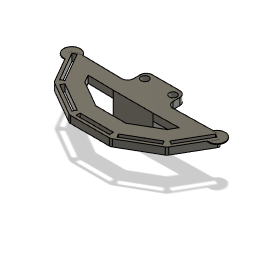
Sensorhållare v11 (Autodesk Fusion 360 design; units mm, degrees)
Autodesk Fusion 360 part; units mm, degrees
note: some values were not read from the file. Set by a fixed rule: which sketch regions a step uses.
sketch "Sketch1" plane through (0, 0, 0) normal (0, 1, 0) x (1, 0, 0)
  line L0 (0, 0) -> (6, 0) construction
  line L1 (0, 0) -> (-6, 0) construction
  circle A0 centre (6, 0) radius 1.6
  circle A1 centre (-6, 0) radius 1.6
  line L2 (0, 0) -> (0, 3) construction
  line L3 (0, 3) -> (-8.4, 3)
  line L4 (-8.4, 3) -> (-8.4, -5)
  line L5 (-8.4, -5) -> (8.4, -5)
  line L6 (8.4, -5) -> (8.4, 3)
  line L7 (8.4, 3) -> (0, 3)
  line L8 (-8, -26.4564) -> (8, -26.4564)
  line L9 (8, -26.4564) -> (21.8564, -18.4564)
  line L10 (-8, -26.4564) -> (-21.8564, -18.4564)
  line L11 (21.8564, -18.4564) -> (8.4, -5) construction
  line L12 (-21.8564, -18.4564) -> (-8.4, -5) construction
  line L13 (21.8564, -18.4564) -> (29.8564, -4.6)
  line L14 (29.8564, -4.6) -> (8.4, -5)
  line L15 (-21.8564, -18.4564) -> (-29.8564, -4.6)
  line L16 (-29.8564, -4.6) -> (-8.4, -5)
  line L17 (-8.4559, -11) -> (8.4559, -11)
  line L18 (19.3504, -10.7969) -> (8.4559, -11)
  line L19 (17.4641, -14.0641) -> (19.3504, -10.7969)
  line L20 (6.3923, -20.4564) -> (17.4641, -14.0641)
  line L21 (-6.3923, -20.4564) -> (6.3923, -20.4564)
  line L22 (-6.3923, -20.4564) -> (-17.4641, -14.0641)
  line L23 (-17.4641, -14.0641) -> (-19.3504, -10.7969)
  line L24 (-19.3504, -10.7969) -> (-8.4559, -11)
  line L25 (-7.1, -28.1064) -> (7.1, -28.1064)
  line L26 (7.1, -26.4564) -> (7.1, -28.1064)
  line L27 (-7.1, -26.4564) -> (-7.1, -28.1064)
  line L28 (-21.077, -18.9064) -> (-21.902, -20.3353)
  line L29 (-21.902, -20.3353) -> (-9.6044, -27.4353)
  line L30 (-9.6044, -27.4353) -> (-8.7794, -26.0064)
  line L31 (-22.3064, -17.677) -> (-23.7353, -18.502)
  line L32 (-23.7353, -18.502) -> (-30.8353, -6.2044)
  line L33 (-30.8353, -6.2044) -> (-29.4064, -5.3794)
  line L34 (29.4064, -5.3794) -> (30.8353, -6.2044)
  line L35 (30.8353, -6.2044) -> (23.7353, -18.502)
  line L36 (23.7353, -18.502) -> (22.3064, -17.677)
  line L37 (8.7794, -26.0064) -> (9.6044, -27.4353)
  line L38 (9.6044, -27.4353) -> (21.902, -20.3353)
  line L39 (21.902, -20.3353) -> (21.077, -18.9064)
  line L40 (0, -28.1064) -> (0, -26.4564) construction
  line L41 (-15.7532, -23.8853) -> (-14.9282, -22.4564) construction
  line L42 (-27.2853, -12.3532) -> (-25.8564, -11.5282) construction
  line L43 (25.8564, -11.5282) -> (27.2853, -12.3532) construction
  line L44 (14.9282, -22.4564) -> (15.7532, -23.8853) construction
  line L45 (23.9794, -20.5794) -> (32.3679, -6.05)
  line L46 (8.7771, -29.3564) -> (23.9794, -20.5794)
  line L47 (-8.7771, -29.3564) -> (8.7771, -29.3564)
  line L48 (-8.7771, -29.3564) -> (-23.9794, -20.5794)
  line L49 (-23.9794, -20.5794) -> (-32.3679, -6.05)
  line L50 (-29.8564, -4.6) -> (-32.3679, -6.05)
  line L51 (32.3679, -6.05) -> (29.8564, -4.6)
  circle A2 centre (6, 0) radius 1.8
  circle A3 centre (-6, 0) radius 1.8
  dimension "d1" = 12
  dimension "d2" = 3.2
  dimension "d4" = 3
  dimension "d5" = 5
  dimension "d7" = 16.8
  dimension "d10" = 135
  dimension "d11" = 135
  dimension "d12" = 30
  dimension "d13" = 16
  dimension "d14" = 26.4564
  dimension "d15" = 60
  dimension "d16" = 6
  dimension "d24" = 14.2
  dimension "d25" = 1.65
  dimension "d26" = -2.9
  dimension "d27" = 3.6
  constraint coincident L0.start L1.start
  constraint horizontal L0
  constraint parallel L0 L1
  constraint equal L0 L1
  constraint coincident L0.end A0.centre
  constraint coincident L1.end A1.centre
  constraint perpendicular L1 L2
  constraint perpendicular L2 L3
  constraint perpendicular L3 L4
  constraint perpendicular L2 L5
  constraint perpendicular L5 L6
  constraint perpendicular L2 L7
  constraint equal L3 L7
  constraint horizontal L8
  constraint equal L11 L12
  constraint equal L9 L10
  constraint equal L8 L9
  constraint equal L14 L16
  constraint equal L13 L15
  constraint equal L10 L15
  constraint horizontal L25
  constraint coincident L8 L26.start
  constraint coincident L8 L27.start
  constraint perpendicular L25 L27
  constraint coincident L10 L28.start
  constraint perpendicular L10 L28
  constraint perpendicular L28 L29
  constraint coincident L10 L30.end
  constraint perpendicular L10 L30
  constraint coincident L15 L31.start
  constraint perpendicular L15 L31
  constraint perpendicular L31 L32
  constraint coincident L15 L33.end
  constraint perpendicular L15 L33
  constraint coincident L13 L34.start
  constraint perpendicular L13 L34
  constraint perpendicular L34 L35
  constraint coincident L13 L36.end
  constraint perpendicular L13 L36
  constraint perpendicular L8 L26
  constraint equal L25 L35
  constraint equal L29 L32
  constraint equal L25 L29
  constraint coincident L9 L37.start
  constraint perpendicular L9 L37
  constraint perpendicular L37 L38
  constraint coincident L9 L39.end
  constraint perpendicular L9 L39
  constraint equal L25 L38
  constraint midpoint L25 L40.start
  constraint midpoint L8 L40.end
  constraint midpoint L29 L41.start
  constraint midpoint L10 L41.end
  constraint midpoint L32 L42.start
  constraint midpoint L15 L42.end
  constraint midpoint L13 L43.start
  constraint midpoint L35 L43.end
  constraint midpoint L9 L44.start
  constraint midpoint L38 L44.end
  constraint perpendicular L13 L43
  constraint perpendicular L9 L44
  constraint perpendicular L8 L40
  constraint perpendicular L10 L41
  constraint perpendicular L15 L42
  constraint equal L27 L33
  constraint equal L27 L28
  constraint equal L27 L37
  constraint equal L27 L36
  constraint perpendicular L13 L51
  constraint concentric A0 A2
  constraint equal A0 A1
  constraint concentric A1 A3
  constraint equal A2 A3
  measures "d1" distance of L0.end L1.end
  measures "d2" diameter of A0
  measures "d4" distance of L0.start L2.end
  measures "d5" distance of L0.start L5
  measures "d7" distance of L4 L6
  measures "d10" angle of L4 L12
  measures "d11" angle of L6 L11
  measures "d12" angle of L5 L9
  measures "d13" distance of L8.start L8.end
  measures "d14" distance of L0.start L8
  measures "d15" angle of L5 L13
  measures "d24" distance of L25.start L25.end
  measures "d25" distance of L25.end L26.start
  measures "d27" diameter of A2
extrude "Extrude1" add sketch "Sketch1" along normal blind 3 contours L3 L4 L5 L6 L7 | L5 L8 L9 L10 L13 L14 L15 L16 | L8 L9 L10 L13 L15 L25 L26 L27 L28 L29 L30 L31 L32 L33 L34 L35 L36 L37 L38 L39 L45 L46 L47 L48 L49 L50 L51 | A2 | A3 makes body 1
sketch "Sketch2" plane through (0, 0, 0) normal (0, -1, 0) x (1, 0, 0)
  line L0 (7.1, 26.4564) -> (-7.1, 26.4564)
  line L1 (-7.1, 26.4564) -> (-7.1, 28.1064)
  line L2 (-7.1, 28.1064) -> (7.1, 28.1064)
  line L3 (7.1, 28.1064) -> (7.1, 26.4564)
  line L4 (8.7794, 26.0064) -> (9.6044, 27.4353)
  line L5 (9.6044, 27.4353) -> (21.902, 20.3353)
  line L6 (21.902, 20.3353) -> (21.077, 18.9064)
  line L7 (21.077, 18.9064) -> (8.7794, 26.0064)
  line L8 (23.7353, 18.502) -> (30.8353, 6.2044)
  line L9 (30.8353, 6.2044) -> (29.4064, 5.3794)
  line L10 (29.4064, 5.3794) -> (22.3064, 17.677)
  line L11 (22.3064, 17.677) -> (23.7353, 18.502)
  line L12 (-22.3064, 17.677) -> (-29.4064, 5.3794)
  line L13 (-29.4064, 5.3794) -> (-30.8353, 6.2044)
  line L14 (-30.8353, 6.2044) -> (-23.7353, 18.502)
  line L15 (-23.7353, 18.502) -> (-22.3064, 17.677)
  circle A0 centre (-6, 0) radius 1.6
  line L16 (-6.3923, 20.4564) -> (6.3923, 20.4564)
  line L17 (6.3923, 20.4564) -> (17.4641, 14.0641)
  line L18 (17.4641, 14.0641) -> (19.3504, 10.7969)
  line L19 (19.3504, 10.7969) -> (8.4559, 11)
  line L20 (8.4559, 11) -> (-8.4559, 11)
  line L21 (-8.4559, 11) -> (-19.3504, 10.7969)
  line L22 (-19.3504, 10.7969) -> (-17.4641, 14.0641)
  line L23 (-17.4641, 14.0641) -> (-6.3923, 20.4564)
  circle A1 centre (6, 0) radius 1.6
  line L24 (-9.6044, 27.4353) -> (-8.7794, 26.0064)
  line L25 (-8.7794, 26.0064) -> (-21.077, 18.9064)
  line L26 (-21.077, 18.9064) -> (-21.902, 20.3353)
  line L27 (-21.902, 20.3353) -> (-9.6044, 27.4353)
  line L28 (8.7771, 29.3564) -> (-8.7771, 29.3564)
  line L29 (-8.7771, 29.3564) -> (-23.9794, 20.5794)
  line L30 (-23.9794, 20.5794) -> (-32.3679, 6.05)
  line L31 (-32.3679, 6.05) -> (-29.8564, 4.6)
  line L32 (-29.8564, 4.6) -> (-8.4, 5)
  line L33 (-8.4, 5) -> (-8.4, -3)
  line L34 (-8.4, -3) -> (8.4, -3)
  line L35 (8.4, -3) -> (8.4, 5)
  line L36 (8.4, 5) -> (29.8564, 4.6)
  line L37 (29.8564, 4.6) -> (32.3679, 6.05)
  line L38 (32.3679, 6.05) -> (23.9794, 20.5794)
  line L39 (23.9794, 20.5794) -> (8.7771, 29.3564)
  line L40 (8.4, 5) -> (8.4559, 11)
  line L41 (-8.4, 5) -> (-8.4559, 11)
  line L42 (-8.4, -1.8) -> (8.4, -1.8)
  circle A2 centre (6, 0) radius 1.8
  circle A3 centre (-6, 0) radius 1.8
  line L43 (8.4, -0.4) -> (-8.4, -0.4)
  line L44 (3.4, -1.8) -> (3.4, -0.4)
  line L45 (-3.4, -1.8) -> (-3.4, -0.4)
  line L46 (8.4, 5) -> (8.4, -3)
  line L47 (-8.4, -3) -> (-8.4, 5)
  line L48 (-8.4, 5) -> (8.4, 5)
  dimension "d28" = 0.4
  dimension "d29" = 5
  dimension "d30" = 5
  constraint coincident L35.end L36.start
  constraint coincident L19.end L20.start
  constraint coincident L32.end L33.start
  constraint coincident L20.end L21.start
  constraint coincident L33 L42.start
  constraint coincident L35 L42.end
  constraint perpendicular L35 L42
  constraint tangent L42 A2
  constraint coincident L35 L43.start
  constraint coincident L33 L43.end
  constraint perpendicular L33 L43
  constraint coincident L42 L44.start
  constraint coincident L43 L44.end
  constraint perpendicular L43 L44
  constraint coincident L42 L45.start
  constraint coincident L43 L45.end
  constraint perpendicular L43 L45
  measures "d28" distance of L43 origin
  measures "d29" distance of L44 L46
  measures "d30" distance of L45 L47
extrude "Extrude4" add sketch "Sketch2" along normal blind 6.2 and the other way blind -4.2 separate body contours A0 A3 L43 | L33 L35 A2 A3 L43 L46 L47 L48 | A1 A2 L43 picked at (-7.7136, -0.2359) picked at (4.2864, -0.2359) makes body 2
extrude "Extrude5" add sketch "Sketch2" along normal blind 11.2 and the other way blind -6.2 separate body contours A0 A3 L43 | L33 L35 A2 A3 L43 L46 L47 L48 | A1 A2 L43 picked at (-7.7136, -0.2359) picked at (4.2864, -0.2359) makes body 3
extrude "Extrude6" add sketch "Sketch2" along normal blind 14.2 and the other way blind -11.2 contours A0 A3 L43 | A0 A3 L43 | L33 L35 A2 A3 L43 L46 L47 L48 | L33 L42 A3 L43 L47 | L42 A3 L43 L45 | L33 L34 L35 L42 L46 L47 | L42 L43 L44 L45 | L42 A2 L43 L44 | A1 A2 L43 | A1 A2 L43 | L35 L42 A2 L43 L46 bodies 3
extrude "Extrude7" add sketch "Sketch2" along normal blind 14.2 contours L20 L40 L41 L48 bodies 1 2 3
sketch "Sketch3" plane through (0, -14.2, 0) normal (0, -1, 0) x (1, 0, 0)
  circle A0 centre (-6, 0) radius 1.6
  circle A1 centre (6, 0) radius 1.6
  line L0 (8.4, 5) -> (8.4559, 11)
  line L1 (8.4559, 11) -> (-8.4559, 11)
  line L2 (-8.4559, 11) -> (-8.4, 5)
  line L3 (-8.4, 5) -> (-8.4, -3)
  line L4 (-8.4, -3) -> (8.4, -3)
  line L5 (8.4, -3) -> (8.4, 5)
  line L6 (-7.6166, 2.8) -> (-9.2332, 0)
  line L7 (-9.2332, 0) -> (-7.6166, -2.8)
  line L8 (-7.6166, -2.8) -> (-4.3834, -2.8)
  line L9 (-4.3834, -2.8) -> (-2.7668, 0)
  line L10 (-2.7668, 0) -> (-4.3834, 2.8)
  line L11 (-4.3834, 2.8) -> (-7.6166, 2.8)
  line L12 (4.3834, 2.8) -> (2.7668, 0)
  line L13 (2.7668, 0) -> (4.3834, -2.8)
  line L14 (4.3834, -2.8) -> (7.6166, -2.8)
  line L15 (7.6166, -2.8) -> (9.2332, 0)
  line L16 (9.2332, 0) -> (7.6166, 2.8)
  line L17 (7.6166, 2.8) -> (4.3834, 2.8)
  line L18 (-4.3834, -2.8) -> (-4.3834, -3)
  line L19 (4.3834, -2.8) -> (4.3834, -3)
  point P0 (-6, 0)
  point P1 (6, 0)
  dimension "d49" = 5.6
  constraint coincident P0 A0.centre
  constraint coincident P1 A1.centre
  constraint horizontal L11
  constraint horizontal L17
  constraint equal L11 L17
  constraint coincident L4 L18.end
  constraint perpendicular L4 L18
  constraint coincident L4 L19.end
  constraint perpendicular L4 L19
  measures "d49" distance of L8 L11
extrude "Extrude8" cut sketch "Sketch3" against normal blind 2 contours L5 L12 L13 L14 L15 L16 L17 | L4 L5 L14 L15 L19 | L3 L6 L7 L8 L9 L10 L11 | L3 L4 L7 L8 L18 bodies 1
fillet "Fillet2" radius 2.5 2 edges at (8.4, 1.5, 5) (-8.4, 1.5, 5) on bodies 1
fillet "Fillet3" radius 2.5 2 edges at (-8.4, 1.5, -3) (8.4, 1.5, -3) on bodies 1
chamfer "Chamfer1" distance 6 angle 45 1 edges at (0, -14.2, 11) on bodies 1
fillet "Fillet4" radius 1 2 edges at (32.3679, 1.5, 6.05) (-32.3679, 1.5, 6.05) on bodies 1
fillet "Fillet5" radius 2 6 edges at (23.9794, 1.5, 20.5794) (8.7771, 1.5, 29.3564) (-8.7771, 1.5, 29.3564) (-23.9794, 1.5, 20.5794) (-29.8564, 1.5, 4.6) (29.8564, 1.5, 4.6) on bodies 1
sketch "Sketch4" plane through (0, 3, 0) normal (0, 1, 0) x (-1, 0, 0)
  arc A0 (-30.3379, 4.878) -> (-29.3006, 4.6104) centre (-29.3379, 6.61) ccw
  line L0 (-29.3006, 4.6104) -> (-10.9466, 4.9525)
  arc A1 (-8.4, 2.453) -> (-10.9466, 4.9525) centre (-10.9, 2.453) ccw
  line L1 (-8.4, 2.453) -> (-8.4, -0.5)
  arc A2 (-8.4, -0.5) -> (-5.9, -3) centre (-5.9, -0.5) ccw
  line L2 (-5.9, -3) -> (5.9, -3)
  arc A3 (5.9, -3) -> (8.4, -0.5) centre (5.9, -0.5) ccw
  line L3 (8.4, -0.5) -> (8.4, 2.453)
  arc A4 (10.9466, 4.9525) -> (8.4, 2.453) centre (10.9, 2.453) ccw
  line L4 (10.9466, 4.9525) -> (29.3006, 4.6104)
  arc A5 (29.3006, 4.6104) -> (30.3379, 4.878) centre (29.3379, 6.61) ccw
  line L5 (30.3379, 4.878) -> (31.5019, 5.55)
  arc A6 (31.5019, 5.55) -> (31.8679, 6.916) centre (31.0019, 6.416) ccw
  line L6 (31.8679, 6.916) -> (24.2473, 20.1153)
  arc A7 (24.2473, 20.1153) -> (23.5153, 20.8473) centre (22.5153, 19.1153) ccw
  line L7 (23.5153, 20.8473) -> (9.2412, 29.0885)
  arc A8 (9.2412, 29.0885) -> (8.2412, 29.3564) centre (8.2412, 27.3564) ccw
  line L8 (8.2412, 29.3564) -> (-8.2412, 29.3564)
  arc A9 (-8.2412, 29.3564) -> (-9.2412, 29.0885) centre (-8.2412, 27.3564) ccw
  line L9 (-9.2412, 29.0885) -> (-23.5153, 20.8473)
  arc A10 (-23.5153, 20.8473) -> (-24.2473, 20.1153) centre (-22.5153, 19.1153) ccw
  line L10 (-24.2473, 20.1153) -> (-31.8679, 6.916)
  arc A11 (-31.8679, 6.916) -> (-31.5019, 5.55) centre (-31.0019, 6.416) ccw
  line L11 (-31.5019, 5.55) -> (-30.3379, 4.878)
  circle A12 centre (-6, 0) radius 1.6
  circle A13 centre (6, 0) radius 1.6
  line L12 (-6.3923, 20.4564) -> (6.3923, 20.4564)
  line L13 (6.3923, 20.4564) -> (17.4641, 14.0641)
  line L14 (17.4641, 14.0641) -> (19.3504, 10.7969)
  line L15 (19.3504, 10.7969) -> (8.4559, 11)
  line L16 (8.4559, 11) -> (-8.4559, 11)
  line L17 (-8.4559, 11) -> (-19.3504, 10.7969)
  line L18 (-19.3504, 10.7969) -> (-17.4641, 14.0641)
  line L19 (-17.4641, 14.0641) -> (-6.3923, 20.4564)
  line L20 (29.4064, 5.3794) -> (22.3064, 17.677)
  line L21 (22.3064, 17.677) -> (23.7353, 18.502)
  line L22 (23.7353, 18.502) -> (30.8353, 6.2044)
  line L23 (30.8353, 6.2044) -> (29.4064, 5.3794)
  line L24 (-30.8353, 6.2044) -> (-23.7353, 18.502)
  line L25 (-23.7353, 18.502) -> (-22.3064, 17.677)
  line L26 (-22.3064, 17.677) -> (-29.4064, 5.3794)
  line L27 (-29.4064, 5.3794) -> (-30.8353, 6.2044)
  line L28 (7.1, 26.4564) -> (-7.1, 26.4564)
  line L29 (-7.1, 26.4564) -> (-7.1, 28.1064)
  line L30 (-7.1, 28.1064) -> (7.1, 28.1064)
  line L31 (7.1, 28.1064) -> (7.1, 26.4564)
  line L32 (8.7794, 26.0064) -> (9.6044, 27.4353)
  line L33 (9.6044, 27.4353) -> (21.902, 20.3353)
  line L34 (21.902, 20.3353) -> (21.077, 18.9064)
  line L35 (21.077, 18.9064) -> (8.7794, 26.0064)
  line L36 (-9.6044, 27.4353) -> (-8.7794, 26.0064)
  line L37 (-8.7794, 26.0064) -> (-21.077, 18.9064)
  line L38 (-21.077, 18.9064) -> (-21.902, 20.3353)
  line L39 (-21.902, 20.3353) -> (-9.6044, 27.4353)
  circle A14 centre (30.8353, 6.2044) radius 3.5
  circle A15 centre (-30.8353, 6.2044) radius 3.5
  dimension "d55" = 7
  constraint coincident L22.end L23.start
  constraint coincident L24.start L27.end
  constraint equal A14 A15
  measures "d55" diameter of A15
extrude "Extrude9" add sketch "Sketch4" against normal blind 0.3 contours A0 L0 L10 A11 L11 A15 | L4 A5 L5 A6 L6 A14 bodies 1
equation "d7 = 16 mm + 0.4 * 2 mm"
equation "d26 = -1.7 mm - 1.2 mm"
equation "d27 = 1.8 * 2 mm"
equation "d35 = 4.2 mm + 2 mm"
equation "d39 = 4.2 mm + 7 mm"
equation "d41 = -4.2 mm - 2 mm"
equation "d43 = 4.2 mm + 10 mm"
equation "d45 = -4.2 mm - 7 mm"
named bodies: "Sensorhållare"
